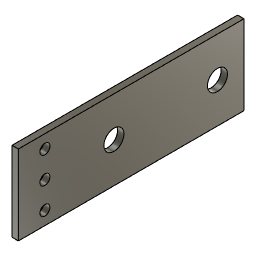
Elevator_TopBracket v1 (Autodesk Fusion 360 design; units mm, degrees)
Autodesk Fusion 360 part; units mm, degrees
sketch "Sketch1" plane through (0, 0, 0) normal (1, 0, 0) x (0, 1, 0)
  line L0 (0, 0) -> (107.95, 0)
  line L1 (107.95, 0) -> (107.95, 38.1)
  line L2 (107.95, 38.1) -> (0, 38.1)
  line L3 (0, 38.1) -> (0, 0)
  dimension "d1" = 38.1
  dimension "d2" = 107.95
  constraint horizontal L0
  constraint vertical L1
  constraint horizontal L2
  constraint vertical L3
  constraint coincident L0.start L3.end
  measures "d1" distance of L0.start L2.end
  measures "d2" distance of L0.start L0.end
extrude "Extrude1" add sketch "Sketch1" along normal blind 3.048
sketch "Sketch2" plane through (3.048, 0, 0) normal (1, 0, 0) x (0, 1, 0)
  line L0 (0, 38.1) -> (0, 0)
  line L1 (0, 0) -> (107.95, 0)
  line L2 (107.95, 0) -> (107.95, 38.1)
  line L3 (107.95, 38.1) -> (0, 38.1)
  line L4 (-12.7, 0) -> (-12.7, 19.05)
  line L5 (0, -12.7) -> (25.4, -12.7)
  line L6 (25.4, -25.4) -> (31.75, -25.4)
  line L7 (33.02, -38.1) -> (45.72, -38.1)
  line L8 (45.72, -50.8) -> (58.42, -50.8)
  line L9 (58.42, -50.8) -> (58.42, -38.1)
  line L10 (58.42, -38.1) -> (71.12, -38.1)
  line L11 (71.12, -38.1) -> (71.12, -50.8)
  line L12 (71.12, -50.8) -> (83.82, -50.8)
  line L13 (83.82, -50.8) -> (83.82, -38.1)
  line L14 (83.82, -38.1) -> (96.52, -38.1)
  line L15 (96.52, -38.1) -> (96.52, -50.8)
  line L16 (96.52, -50.8) -> (109.22, -50.8)
  line L17 (109.22, -50.8) -> (109.22, -38.1)
  line L18 (-12.7, 19.05) -> (121.92, 19.05)
  circle A0 centre (45.72, 19.05) radius 4.826
  dimension "d5" = 19.05
  dimension "d6" = 6.35
  dimension "d7" = 9.652
  constraint perpendicular L1 L4
  constraint horizontal L5
  constraint perpendicular L0 L6
  constraint horizontal L7
  constraint parallel L7 L8
  constraint perpendicular L8 L9
  constraint perpendicular L9 L10
  constraint perpendicular L10 L11
  constraint perpendicular L11 L12
  constraint perpendicular L12 L13
  constraint horizontal L14
  constraint perpendicular L14 L15
  constraint perpendicular L15 L16
  constraint perpendicular L1 L17
  constraint perpendicular L2 L18
  constraint coincident L18 A0.centre
  measures "d5" distance of L4.start L4.end
  measures "d6" distance of L6.start L6.end
  measures "d7" diameter of A0
hole "Hole1" at (3.048, 45.72, 19.05) direction (-1, 0, 0) diameter 9.652 depth 40.64 tip angle 118
sketch "Sketch3" plane through (3.048, 0, 0) normal (1, 0, 0) x (0, 1, 0)
  circle A0 centre (45.72, 19.05) radius 4.826
  line L0 (0, 38.1) -> (0, 0)
  line L1 (0, 0) -> (107.95, 0)
  line L2 (107.95, 0) -> (107.95, 38.1)
  line L3 (107.95, 38.1) -> (0, 38.1)
  line L4 (111.76, 0) -> (111.76, 19.05)
  circle A1 centre (95.25, 19.0673) radius 4.826
  dimension "d16" = 9.652
  constraint parallel L2 L4
  measures "d16" diameter of A1
hole "Hole2" at (3.048, 95.25, 19.0673) direction (-1, 0, 0) diameter 9.652 depth 40.64 tip angle 118
sketch "Sketch4" plane through (3.048, 0, 0) normal (1, 0, 0) x (0, 1, 0)
  circle A0 centre (95.25, 19.0673) radius 4.826
  circle A1 centre (45.72, 19.05) radius 4.826
  line L0 (0, 38.1) -> (0, 0)
  line L1 (0, 0) -> (107.95, 0)
  line L2 (107.95, 0) -> (107.95, 38.1)
  line L3 (107.95, 38.1) -> (0, 38.1)
  line L4 (12.7, -55.88) -> (0, -55.88)
  line L5 (0, -55.88) -> (0, 45.72)
  line L6 (12.7, 0) -> (-25.4, 0)
  line L7 (0, 0) -> (12.7, 0)
  line L8 (12.7, 0) -> (12.7, 6.35)
  line L9 (12.7, 6.35) -> (0, 6.35)
  line L10 (0, 6.35) -> (0, 0)
  dimension "d22" = 12.7
  dimension "d23" = 6.35
  constraint horizontal L4
  constraint vertical L5
  constraint horizontal L6
  constraint coincident L1 L6.start
  constraint horizontal L7
  constraint vertical L8
  constraint horizontal L9
  constraint vertical L10
  constraint coincident L0.end L1.start
  measures "d22" distance of L0.end L6.start
  measures "d23" distance of L0.end L9.end
hole "Hole3" at (3.048, 12.7, 6.35) direction (-1, 0, 0) diameter 4.826 depth 40.64 tip angle 118
sketch "Sketch5" plane through (3.048, 0, 0) normal (1, 0, 0) x (0, 1, 0)
  circle A0 centre (12.7, 6.35) radius 2.413
  circle A1 centre (95.25, 19.0673) radius 4.826
  circle A2 centre (45.72, 19.05) radius 4.826
  line L0 (0, 38.1) -> (0, 0)
  line L1 (0, 0) -> (107.95, 0)
  line L2 (107.95, 0) -> (107.95, 38.1)
  line L3 (107.95, 38.1) -> (0, 38.1)
  line L4 (0, 38.1) -> (12.7, 38.1)
  line L5 (12.7, 38.1) -> (12.7, 31.75)
  line L6 (12.7, 31.75) -> (0, 31.75)
  line L7 (0, 31.75) -> (0, 38.1)
  dimension "d27" = 12.7
  dimension "d28" = 6.35
  constraint horizontal L4
  constraint vertical L5
  constraint horizontal L6
  constraint vertical L7
  constraint coincident L0.start L3.end
  measures "d27" distance of L0.start L4.end
  measures "d28" distance of L0.start L6.end
hole "Hole4" at (3.048, 12.7, 31.75) direction (-1, 0, 0) diameter 4.826 depth 40.64 tip angle 118
sketch "Sketch6" plane through (3.048, 0, 0) normal (1, 0, 0) x (0, 1, 0)
  circle A0 centre (12.7, 31.75) radius 2.413
  circle A1 centre (12.7, 6.35) radius 2.413
  circle A2 centre (95.25, 19.0673) radius 4.826
  circle A3 centre (45.72, 19.05) radius 4.826
  line L0 (0, 38.1) -> (0, 0)
  line L1 (0, 0) -> (107.95, 0)
  line L2 (107.95, 0) -> (107.95, 38.1)
  line L3 (107.95, 38.1) -> (0, 38.1)
  line L4 (0, 0) -> (12.7, 0)
  line L5 (12.7, 0) -> (12.7, 19.05)
  line L6 (12.7, 19.05) -> (0, 19.05)
  line L7 (0, 19.05) -> (0, 0)
  dimension "d32" = 12.7
  dimension "d33" = 19.05
  constraint horizontal L4
  constraint vertical L5
  constraint horizontal L6
  constraint vertical L7
  constraint coincident L0.end L1.start
  measures "d32" distance of L0.end L4.end
  measures "d33" distance of L0.end L6.end
hole "Hole5" at (3.048, 12.7, 19.05) direction (-1, 0, 0) diameter 4.826 depth 40.64 tip angle 118
